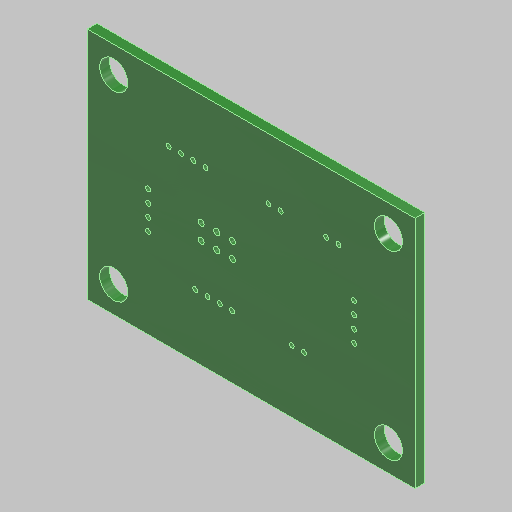
# Autodesk Inventor part: board
Saved by Autodesk Inventor 2023.5 (Build 275446000, 446)
## iProperties
Created: 2024-02-02
Part Number: board
Material: Generic
Document SubType Name: Modeling
Designer: Paul
Density: 1 g/cm^3
Appearance: Forest Green
Mass: 3.12884 g
Surface Area: 43.8405 cm^2
Volume: 3.12884 cm^3
Author: Paul
Autodesk Inventor part; units mm, degrees
ref_plane "YZ Plane" through (0, 0, 0) normal (1, 0, 0) x (0, 1, 0)
ref_plane "XZ Plane" through (0, 0, 0) normal (0, 1, 0) x (-1, 0, 0)
ref_plane "XY Plane" through (0, 0, 0) normal (0, 0, 1) x (1, 0, 0)
sketch "Sketch1" plane through (0, 0, 0) normal (0, 0, 1) x (1, 0, 0)
  line L0 (0, 0) -> (53.34, 0)
  line L1 (53.34, 0) -> (53.34, 38.1)
  line L2 (53.34, 38.1) -> (0, 38.1)
  line L3 (0, 38.1) -> (0, 0)
  dimension "d0" = 53.34
  dimension "d1" = 38.1
  constraints: 8 end point, 2 parallel, 1 horizontal, 1 perpendicular
  measures "d0" distance of L1.end L2.end
  measures "d1" distance of L2.end L0.start
extrude "Extrusion1" add sketch "Sketch1" along normal blind 1.6
sketch "Sketch2" plane through (0, 0, 1.6) normal (0, 0, 1) x (1, 0, 0)
  line L0 (53.34, 38.1) -> (0, 38.1) projected
  line L1 (0, 0) -> (53.34, 0) projected
  line L2 (0, 38.1) -> (0, 0) projected
  line L3 (53.34, 0) -> (53.34, 38.1) projected
  point P0 (4.318, 33.782)
  point P1 (49.022, 33.782)
  point P2 (49.022, 4.318)
  point P3 (4.318, 4.318)
  dimension "d4" = 29.464
  dimension "d5" = 4.318
  dimension "d6" = 38.1
  dimension "d7" = 53.34
  dimension "d8" = 4.318
  dimension "d9" = 4.318
  constraints: 2 horizontal alignment, 2 vertical alignment
  measures "d4" distance of point (49.022, 4.318) point (49.022, 33.782)
  measures "d5" distance from line of L0 point (49.022, 33.782)
  measures "d6" distance between parallel lines of L0 L1
  measures "d7" distance between parallel lines of L2 L3
  measures "d8" distance from line of L3 point (49.022, 33.782)
  measures "d9" distance from line of L2 point (4.318, 33.782)
hole "Hole1" at (4.318, 33.782, 1.6) at (49.022, 33.782, 1.6) at (49.022, 4.318, 1.6) at (4.318, 4.318, 1.6) direction (0, 0, -1) diameter 4.572 end through all
sketch "Sketch3" plane through (0, 0, 1.6) normal (0, 0, 1) x (1, 0, 0)
  line L0 (0, 38.1) -> (0, 0) projected
  line L1 (53.34, 38.1) -> (0, 38.1) projected
  line L2 (0, 0) -> (53.34, 0) projected
  line L3 (53.34, 0) -> (53.34, 38.1) projected
  point P0 (19.256, 28.194)
  point P1 (31.48, 28.194)
  point P2 (40.878, 28.194)
  point P3 (9.921, 20.526)
  point P4 (43.419, 15.542)
  point P5 (17.574, 10.175)
  point P6 (33.29, 10.175)
  point P7 (17.256, 28.194)
  point P8 (15.256, 28.194)
  point P9 (13.256, 28.194)
  point P10 (38.878, 28.194)
  point P11 (29.48, 28.194)
  point P12 (9.921, 18.526)
  point P13 (9.921, 16.526)
  point P14 (9.921, 14.526)
  point P15 (19.574, 10.175)
  point P16 (21.574, 10.175)
  point P17 (23.574, 10.175)
  point P18 (35.29, 10.175)
  point P19 (43.419, 17.542)
  point P20 (43.419, 19.542)
  point P21 (43.419, 21.542)
  dimension "d17" = 19.256
  dimension "d18" = 31.48
  dimension "d19" = 40.878
  dimension "d20" = 9.906
  dimension "d44" = 2
  dimension "d51" = 2
  dimension "d58" = 2
  dimension "d63" = 9.921
  dimension "d64" = 17.574
  dimension "d65" = 17.574
  dimension "d66" = 10.175
  dimension "d67" = 33.29
  dimension "d68" = 15.542
  dimension "d69" = 9.921
  dimension "d72" = 2
  dimension "d79" = 2
  dimension "d86" = 2
  dimension "d93" = 2
  constraints: 5 horizontal, 3 horizontal alignment, 2 vertical, 15 other
  measures "d17" distance from line of L0 point (19.256, 28.194)
  measures "d18" distance from line of L0 point (31.48, 28.194)
  measures "d19" distance from line of L0 point (40.878, 28.194)
  measures "d20" distance from line of L1 point (19.256, 28.194)
  measures "d44" distance of point (19.256, 28.194) point (17.256, 28.194)
  measures "d51" distance of point (40.878, 28.194) point (38.878, 28.194)
  measures "d58" distance of point (31.48, 28.194) point (29.48, 28.194)
  measures "d63" distance from line of L0 point (9.921, 20.526)
  measures "d64" distance from line of L1 point (9.921, 20.526)
  measures "d65" distance from line of L0 point (17.574, 10.175)
  measures "d66" vertical distance of L0.end point (17.574, 10.175)
  measures "d67" distance from line of L0 point (33.29, 10.175)
  measures "d68" distance from line of L2 point (43.419, 15.542)
  measures "d69" distance from line of L3 point (43.419, 15.542)
  measures "d72" distance of point (9.921, 20.526) point (9.921, 18.526)
  measures "d79" distance of point (17.574, 10.175) point (19.574, 10.175)
  measures "d86" distance of point (33.29, 10.175) point (35.29, 10.175)
  measures "d93" distance of point (43.419, 15.542) point (43.419, 17.542)
hole "Hole2" at (19.256, 28.194, 1.6) at (31.48, 28.194, 1.6) at (40.878, 28.194, 1.6) at (9.921, 20.526, 1.6) at (43.419, 15.542, 1.6) at (17.574, 10.175, 1.6) at (33.29, 10.175, 1.6) at (17.256, 28.194, 1.6) at (15.256, 28.194, 1.6) at (13.256, 28.194, 1.6) at (38.878, 28.194, 1.6) at (29.48, 28.194, 1.6) at (9.921, 18.526, 1.6) at (9.921, 16.526, 1.6) at (9.921, 14.526, 1.6) at (19.574, 10.175, 1.6) at (21.574, 10.175, 1.6) at (23.574, 10.175, 1.6) at (35.29, 10.175, 1.6) at (43.419, 17.542, 1.6) at (43.419, 19.542, 1.6) at (43.419, 21.542, 1.6) direction (0, 0, -1) diameter 0.8 end through all
sketch "Sketch4" plane through (0, 0, 1.6) normal (0, 0, 1) x (1, 0, 0)
  line L0 (53.34, 38.1) -> (0, 38.1) projected
  line L1 (0, 38.1) -> (0, 0) projected
  point P0 (18.557, 17.521)
  point P1 (21.097, 17.521)
  point P2 (23.637, 17.521)
  point P3 (18.557, 20.061)
  point P4 (21.097, 20.061)
  point P5 (23.637, 20.061)
  dimension "d105" = 20.579
  dimension "d106" = 18.557
  dimension "d109" = 2.54
  dimension "d112" = 2.54
  constraints: 1 horizontal, 1 vertical, 5 other
  measures "d105" distance from line of L0 point (18.557, 17.521)
  measures "d106" distance from line of L1 point (18.557, 17.521)
  measures "d109" distance of point (18.557, 17.521) point (21.097, 17.521)
  measures "d112" distance of point (18.557, 17.521) point (18.557, 20.061)
hole "Hole3" at (18.557, 17.521, 1.6) at (21.097, 17.521, 1.6) at (23.637, 17.521, 1.6) at (18.557, 20.061, 1.6) at (21.097, 20.061, 1.6) at (23.637, 20.061, 1.6) direction (0, 0, -1) diameter 1 end through all
equation "\"d5\" = -0.5 * d4 + 0.5 * d6"
equation "\"d8\" = d5"
equation "\"d9\" = d5"
body "Solid1"
